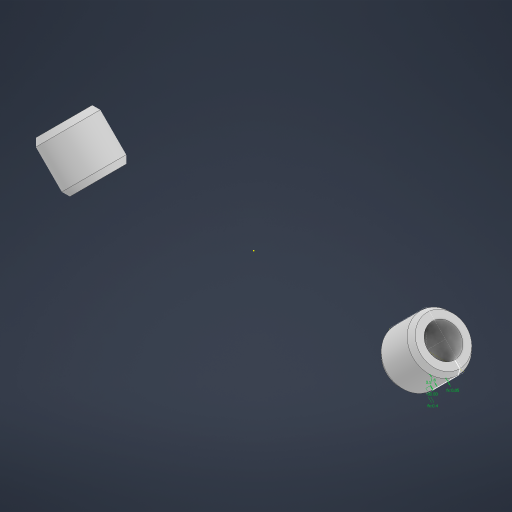
# Autodesk Inventor part: Slew Bearing
Saved by Autodesk Inventor 2023.1 (Build 271208000, 208)
## iProperties
Created: 2022-11-26
Part Number: Slew Bearing
Material: Generic
Document SubType Name: Modeling
Designer: aubrey-work
Density: 1 g/cm^3
Appearance: Default
Author: aubrey-work
Autodesk Inventor part; units mm, degrees
ref_plane "YZ Plane" through (0, 0, 0) normal (1, 0, 0) x (0, 1, 0)
ref_plane "XZ Plane" through (0, 0, 0) normal (0, 1, 0) x (-1, 0, 0)
ref_plane "XY Plane" through (0, 0, 0) normal (0, 0, 1) x (1, 0, 0)
sketch "Sketch1" plane through (0, 0, 0) normal (0, 1, 0) x (-1, 0, 0)
  circle A0 centre (0, 0) radius 26.2043 construction
  ellipse E0 centre (-26.2043, 0) end of major axis (-31.9319, 0) minor radius 4.05 construction
  line L0 (-31.9319, 0) -> (26.2043, 0) construction
  line L1 (-31.9319, 0) -> (-20.4767, 0) construction
  line L2 (0, 0) -> (-24.9524, -3.9521) construction
  dimension "d0" = 5.7276
  dimension "d1" = 4.05
  dimension "d2" = 9
  constraints: 6 end point, 3 point on line, 2 point on circle, 1 centre point, 1 coincident, 1 horizontal, 6 other
  measures "d2" angle of L0 L2
sketch "Sketch2" plane through (0, 0, 0) normal (0, 0, 1) x (1, 0, 0)
  line L0 (31.9319, 0) -> (20.4767, 0) construction
  line L1 (20.4767, 0) -> (26.2043, -5.7276) construction
  line L2 (26.2043, -5.7276) -> (31.9319, 0) construction
  line L3 (20.4767, 0) -> (26.2043, 5.7276) construction
  line L4 (26.2043, 5.7276) -> (31.9319, 0) construction
  line L5 (29.0681, 2.8638) -> (23.3405, -2.8638) construction
  line L6 (29.0681, -2.8638) -> (23.3405, 2.8638) construction
  line L7 (26.2043, -5.7276) -> (26.2043, 5.7276) construction
  line L8 (25.3204, -4.278) -> (30.4823, 0.8839)
  line L9 (30.4823, 0.8839) -> (31.2601, 0.1061)
  line L10 (31.2601, 0.1061) -> (31.0013, -0.8599)
  line L11 (31.0013, -0.8599) -> (27.0642, -4.797)
  line L12 (27.0642, -4.797) -> (26.0982, -5.0558)
  line L13 (26.0982, -5.0558) -> (25.3204, -4.278)
  point P0 (0, 0)
  dimension "d3" = 0.05
  dimension "d4" = 0.4
  dimension "d5" = 60
  dimension "d7" = 1.6
  dimension "d9" = 0.5
  constraints: 26 end point, 4 midpoint, 4 symmetric about line, 3 perpendicular, 2 parallel
  measures "d3" distance between parallel lines of L2 L11
  measures "d4" distance between parallel lines of L1 L13
  measures "d5" angle of L13 L12
  measures "d7" distance between parallel lines of L11 L8
  measures "d9" distance from line of L12.end L11
revolve "Revolution1" add sketch "Sketch2" angle 360 about axis through (29.0681, 2.8638, 0) along (-0.7071068, -0.7071068, 0)
mirror "Mirror1" about plane through (0, 0, 0) normal (1, 0, 0)
equation "\"d0\" = 1.41421 * d1"
equation "\"d1\" = 0.5 * gap + 0.5 * roller_outerDiameter"
equation "\"d3\" = 0.5 * gap"
equation "\"d4\" = airgap"
equation "\"gap\" = 0.1"
equation "\"roller_outerDiameter\" = 8"
equation "\"wallgap\" = 2"
equation "\"airgap\" = 0.4"
body "Solid1"
